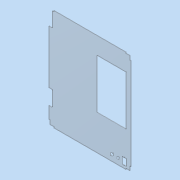
# Autodesk Inventor part: 101.003.01_Abdeckung_HMI_links
Saved by Autodesk Inventor 2022 (Build 260153000, 153)
## iProperties
Created: 2021-11-25
Part Number: 101.003.01_Abdeckung_HMI_links
Material: PMMA-Kunststoff
Document SubType Name: Modeling
Designer: Sebastian Seewald
Mass: 65.5279 g
Surface Area: 298.591 cm^2
Volume: 55.1582 cm^3
Density: 1.188 g/cm^3
Appearance: Polycarbonat - klar
Author: Sebastian Seewald
Autodesk Inventor part; units mm, degrees
ref_plane "YZ Plane" through (0, 0, 0) normal (1, 0, 0) x (0, 1, 0)
ref_plane "XZ Plane" through (0, 0, 0) normal (0, 1, 0) x (-1, 0, 0)
ref_plane "XY Plane" through (0, 0, 0) normal (0, 0, 1) x (1, 0, 0)
sketch "Skizze1" plane through (0, 0, 0) normal (0, 0, 1) x (1, 0, 0)
  line L0 (0, 0) -> (662.5, 0)
  line L1 (662.5, 0) -> (662.5, 822.5)
  line L2 (662.5, 822.5) -> (0, 822.5)
  line L3 (0, 822.5) -> (0, 0)
  line L4 (0, 822.5) -> (40, 822.5)
  line L5 (40, 822.5) -> (40, 814.5)
  line L6 (40, 814.5) -> (0, 814.5)
  line L7 (0, 814.5) -> (0, 822.5)
  line L8 (0, 822.5) -> (8, 822.5)
  line L9 (8, 822.5) -> (8, 782.5)
  line L10 (8, 782.5) -> (0, 782.5)
  line L11 (0, 782.5) -> (0, 822.5)
  line L12 (0, 411.25) -> (662.5, 411.25) construction
  line L13 (331.25, 822.5) -> (331.25, 0) construction
  line L14 (0, 0) -> (40, 0)
  line L15 (40, 0) -> (40, 8)
  line L16 (40, 8) -> (0, 8)
  line L17 (0, 8) -> (0, 0)
  line L18 (0, 0) -> (8, 0)
  line L19 (8, 0) -> (8, 40)
  line L20 (8, 40) -> (0, 40)
  line L21 (0, 40) -> (0, 0)
  line L22 (662.5, 822.5) -> (662.5, 0)
  line L23 (662.5, 822.5) -> (622.5, 822.5)
  line L24 (622.5, 822.5) -> (622.5, 814.5)
  line L25 (622.5, 814.5) -> (662.5, 814.5)
  line L26 (662.5, 814.5) -> (662.5, 822.5)
  line L27 (662.5, 822.5) -> (654.5, 822.5)
  line L28 (654.5, 822.5) -> (654.5, 782.5)
  line L29 (654.5, 782.5) -> (662.5, 782.5)
  line L30 (662.5, 782.5) -> (662.5, 822.5)
  line L31 (662.5, 0) -> (654.5, 0)
  line L32 (662.5, 0) -> (622.5, 0)
  line L33 (622.5, 0) -> (622.5, 8)
  line L34 (622.5, 8) -> (662.5, 8)
  line L35 (654.5, 0) -> (654.5, 40)
  line L36 (662.5, 8) -> (662.5, 0)
  line L37 (654.5, 40) -> (662.5, 40)
  line L38 (662.5, 40) -> (662.5, 0)
  point P0 (662.5, 782.5)
  point P1 (654.5, 814.5)
  point P2 (8, 814.5)
  point P3 (0, 782.5)
  point P4 (0, 40)
  point P5 (8, 8)
  point P6 (654.5, 8)
  point P7 (662.5, 40)
  dimension "d0" = 662.5
  dimension "d1" = 822.5
  dimension "d2" = 40
  dimension "d3" = 8
  dimension "d4" = 8
  dimension "d5" = 40
  constraints: 78 end point, 18 symmetric about line, 6 parallel, 4 midpoint, 3 horizontal, 3 perpendicular
  measures "d0" distance of L1.end L2.end
  measures "d1" distance between parallel lines of L0 L2
  measures "d2" distance between parallel lines of L3 L5
  measures "d3" distance between parallel lines of L2 L6
  measures "d4" distance between parallel lines of L3 L9
  measures "d5" distance between parallel lines of L2 L10
extrude "Extrusion1" add sketch "Skizze1" along normal blind 4 contours L15 L16 L19 L20 L3 L10 L9 L6 L5 L2 L24 L25 L28 L29 L1 L37 L35 L34 L33 L0
sketch "Skizze2" plane through (0, 0, 0) normal (0, 0, -1) x (-1, 0, 0)
  line L0 (-624.5, 683.3) -> (-389.5, 683.3)
  line L1 (-389.5, 683.3) -> (-389.5, 284.3)
  line L2 (-389.5, 284.3) -> (-624.5, 284.3)
  line L3 (-624.5, 284.3) -> (-624.5, 683.3)
  line L4 (-654.5, 782.5) -> (-654.5, 814.5) projected
  line L5 (-654.5, 814.5) -> (-622.5, 814.5) projected
  point P0 (0, 0)
  dimension "d11" = 399
  dimension "d12" = 235
  dimension "d13" = 30
  dimension "d14" = 131.2
  constraints: 8 end point, 2 parallel, 1 horizontal, 1 perpendicular
  measures "d11" distance between parallel lines of L2 L0
  measures "d12" distance between parallel lines of L3 L1
  measures "d13" distance between parallel lines of L3 L4
  measures "d14" distance between parallel lines of L0 L5
extrude "Extrusion2" cut sketch "Skizze2" against normal up to surface (4 mm away)
sketch "Skizze3" plane through (0, 0, 0) normal (0, 0, -1) x (-1, 0, 0)
  line L0 (0, 782.5) -> (0, 40) projected
  line L1 (-28, 814.5) -> (0, 814.5)
  line L2 (0, 814.5) -> (0, 694.5)
  line L3 (0, 694.5) -> (-23, 694.5)
  line L4 (-28, 699.5) -> (-28, 814.5)
  line L5 (0, 263) -> (-23, 263)
  line L6 (-28, 258) -> (-28, 143)
  line L7 (-23, 138) -> (0, 138)
  line L8 (0, 138) -> (0, 263)
  line L9 (-8, 40) -> (-8, 8) projected
  line L10 (-8, 8) -> (-40, 8) projected
  line L11 (-8, 814.5) -> (-8, 782.5) projected
  line L12 (-40, 814.5) -> (-8, 814.5) projected
  arc A0 (-28, 699.5) -> (-23, 694.5) centre (-23, 699.5) ccw
  arc A1 (-23, 263) -> (-28, 258) centre (-23, 258) ccw
  arc A2 (-28, 143) -> (-23, 138) centre (-23, 143) ccw
  point P0 (0, 0)
  point P1 (-28, 694.5)
  point P2 (-28, 263)
  point P3 (0, 138)
  point P4 (0, 686.15)
  point P5 (-28, 138)
  point P6 (0, 138)
  dimension "d17" = 20
  dimension "d19" = 20
  dimension "d20" = 0
  dimension "d21" = 120
  dimension "d61" = 130
  dimension "d62" = 120
  dimension "d63" = 5
  dimension "d64" = 5
  constraints: 18 end point, 8 point on line, 6 point on circle, 6 tangent, 4 parallel, 3 centre point, 2 horizontal, 2 perpendicular
  measures "d17" distance between parallel lines of L9 L6
  measures "d19" distance between parallel lines of L4 L11
  measures "d20" distance between parallel lines of L12 L1
  measures "d21" distance between parallel lines of L1 L3
  measures "d61" distance between parallel lines of L10 L7
  measures "d62" distance of L6.start point (-28, 138)
  measures "d63" radius of A2
  measures "d64" radius of A1
extrude "Extrusion3" cut sketch "Skizze3" against normal up to surface (4 mm away)
sketch "Skizze4" plane through (0, 0, 0) normal (0, 0, -1) x (-1, 0, 0)
  line L0 (-619.5, 194.3) -> (-449.5, 194.3)
  line L1 (-444.5, 189.3) -> (-444.5, 159.3)
  line L2 (-449.5, 154.3) -> (-619.5, 154.3)
  line L3 (-624.5, 159.3) -> (-624.5, 189.3)
  line L4 (-624.5, 284.3) -> (-624.5, 683.3) projected
  line L5 (-389.5, 284.3) -> (-624.5, 284.3) projected
  arc A0 (-619.5, 194.3) -> (-624.5, 189.3) centre (-619.5, 189.3) ccw
  arc A1 (-624.5, 159.3) -> (-619.5, 154.3) centre (-619.5, 159.3) ccw
  arc A2 (-449.5, 154.3) -> (-444.5, 159.3) centre (-449.5, 159.3) ccw
  arc A3 (-444.5, 189.3) -> (-449.5, 194.3) centre (-449.5, 189.3) ccw
  point P0 (0, 0)
  dimension "d25" = 90
  dimension "d26" = 40
  dimension "d27" = 180
  dimension "d28" = 5
  constraints: 8 end point, 8 point on circle, 8 tangent, 4 centre point, 3 equal radius, 2 parallel, 1 collinear, 1 horizontal, 1 perpendicular
  measures "d25" distance between parallel lines of L0 L5
  measures "d26" distance between parallel lines of L0 L2
  measures "d27" distance between parallel lines of L3 L1
  measures "d28" radius of A0
extrude "Extrusion4" cut sketch "Skizze4" against normal up to surface (4 mm away)
sketch "Skizze5" plane through (0, 0, 0) normal (0, 0, -1) x (-1, 0, 0)
  line L0 (-645.9539, 213.8422) -> (-402.4483, 213.8422)
  line L1 (-402.4483, 213.8422) -> (-402.4483, 126.1802)
  line L2 (-402.4483, 126.1802) -> (-645.9539, 126.1802)
  line L3 (-645.9539, 126.1802) -> (-645.9539, 213.8422)
  point P0 (0, 0)
  constraints: 8 end point, 2 parallel, 1 horizontal, 1 perpendicular
extrude "Extrusion5" add sketch "Skizze5" against normal blind 4
sketch "Skizze6" plane through (0, 0, 0) normal (0, 0, -1) x (-1, 0, 0)
  line L0 (-625.2, 76.6) -> (-592.2, 76.6)
  line L1 (-592.2, 76.6) -> (-592.2, 23.4)
  line L2 (-592.2, 23.4) -> (-625.2, 23.4)
  line L3 (-625.2, 23.4) -> (-625.2, 76.6)
  circle A0 centre (-608.7, 79.25) radius 1.7
  circle A1 centre (-608.7, 20.75) radius 1.7
  line L4 (-40, 0) -> (-622.5, 0) projected
  line L5 (-662.5, 40) -> (-662.5, 782.5) projected
  arc A2 (-567.7, 44.7885) -> (-567.7, 55.2115) centre (-558.7, 50) ccw
  line L6 (-567.7, 55.2115) -> (-567.7, 44.7885)
  circle A3 centre (-508.7, 50) radius 11.8
  circle A4 centre (-518.2, 62) radius 1.75
  circle A5 centre (-499.2, 38) radius 1.75
  line L7 (-654.7, 10) -> (-654.7, 0) construction
  line L8 (-654.5, 8) -> (-654.5, 40) projected
  point P0 (0, 0)
  point P1 (-592.2, 50)
  point P2 (-625.2, 50)
  point P3 (-608.7, 23.4)
  dimension "d33" = 53.2
  dimension "d34" = 33
  dimension "d35" = 16.5
  dimension "d36" = 0
  dimension "d37" = 58.5
  dimension "d38" = 29.25
  dimension "d39" = 3.4
  dimension "d40" = 50
  dimension "d43" = 20.8
  dimension "d44" = 19.4
  dimension "d45" = 0
  dimension "d46" = 50
  dimension "d47" = 24
  dimension "d48" = 12
  dimension "d49" = 23.6
  dimension "d50" = 19
  dimension "d51" = 9.5
  dimension "d52" = 3.5
  dimension "d53" = 0
  dimension "d54" = 50
  dimension "d55" = 10
  dimension "d56" = 0
  dimension "d57" = 0.2
  dimension "d58" = 46
  constraints: 12 end point, 6 centre point, 3 midpoint, 2 equal radius, 2 parallel, 2 point on circle, 2 vertical, 1 horizontal, 1 perpendicular
  measures "d33" distance of L0.end L1.end
  measures "d34" distance of L0.start L0.end
  measures "d35" distance from line of A0.centre L3
  measures "d36" horizontal distance of A1.centre A0.centre
  measures "d37" distance of A0.centre A1.centre
  measures "d38" vertical distance of point (-592.2, 50) A0.centre
  measures "d39" diameter of A0
  measures "d40" distance from line of L4 point (-625.2, 50)
  measures "d43" diameter of A2
  measures "d45" vertical distance of point (-592.2, 50) A2.centre
  measures "d46" horizontal distance of point (-608.7, 23.4) A2.centre
  measures "d47" vertical distance of A5.centre A4.centre
  measures "d48" vertical distance of A5.centre A3.centre
  measures "d49" diameter of A3
  measures "d50" horizontal distance of A4.centre A5.centre
  measures "d51" horizontal distance of A3.centre A4.centre
  measures "d52" diameter of A5
  measures "d53" vertical distance of A3.centre A2.centre
  measures "d54" distance of A3.centre A2.centre
  measures "d55" distance of L7.start L7.end
  measures "d56" vertical distance of point (0, 0) L7.end
  measures "d57" distance between parallel lines of L7 L8
  measures "d58" distance from line of A1.centre L7
extrude "Extrusion6" cut sketch "Skizze6" against normal blind 4
equation "\"d35\" = 0.5 * d34"
equation "\"d38\" = 0.5 * d37"
equation "\"d48\" = 0.5 * d47"
equation "\"d51\" = 0.5 * d50"
equation "\"d54\" = d46"
